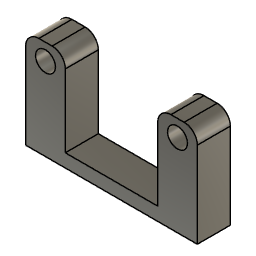
sumobot_base v24 (Autodesk Fusion 360 archive; units mm, degrees)
design "lidar_mount"
Autodesk Fusion 360 part; units mm, degrees
sketch "Sketch1" plane through (0, 0, 0) normal (0, 0, 1) x (1, 0, 0)
  line L0 (13, 2) -> (-13, 2)
  line L1 (-13, 2) -> (-13, -2)
  line L2 (-13, -2) -> (13, -2)
  line L3 (13, -2) -> (13, 2)
  line L4 (13, 2) -> (-13, -2) construction
  line L5 (-13, 2) -> (13, -2) construction
  dimension "d1" = 26
  dimension "d2" = 4
  constraint horizontal L0
  constraint perpendicular L0 L1
  constraint parallel L0 L2
  constraint parallel L1 L3
  constraint coincident L4 origin
  constraint coincident L5 origin
  measures "d1" distance of L1.end L2.end
  measures "d2" distance of L0.end L1.end
extrude "Extrude1" add sketch "Sketch1" along normal blind 2
sketch "Sketch2" plane through (0, 0, 2) normal (0, 0, 1) x (-1, 0, 0)
  line L0 (-13, 2) -> (-13, -2)
  line L1 (-13, -2) -> (13, -2)
  line L2 (13, -2) -> (13, 2)
  line L3 (13, 2) -> (-13, 2)
  line L4 (13, -2) -> (7, -2)
  line L5 (7, -2) -> (7, 2)
  line L6 (7, 2) -> (13, 2)
  line L7 (13, 2) -> (13, -2)
  line L8 (-13, -2) -> (-7, -2)
  line L9 (-7, -2) -> (-7, 2)
  line L10 (-7, 2) -> (-13, 2)
  line L11 (-13, 2) -> (-13, -2)
  constraint horizontal L4
  constraint vertical L5
  constraint horizontal L6
  constraint vertical L7
  constraint coincident L3 L5.end
  constraint coincident L1.end L2.start
  constraint horizontal L8
  constraint vertical L9
  constraint horizontal L10
  constraint vertical L11
  constraint coincident L3 L9.end
  constraint coincident L0.end L1.start
extrude "Extrude2" add sketch "Sketch2" along normal blind 13 contours L0 L1 L3 L8 L9 L10 L11 | L1 L2 L3 L4 L5 L6 L7
sketch "Sketch3" plane through (0, -2, 0) normal (0, -1, 0) x (1, 0, 0)
  line L0 (-13, 0) -> (13, 0)
  line L1 (13, 0) -> (13, 15)
  line L2 (13, 15) -> (7, 15)
  line L3 (7, 15) -> (7, 2)
  line L4 (7, 2) -> (-7, 2)
  line L5 (-7, 2) -> (-7, 15)
  line L6 (-7, 15) -> (-13, 15)
  line L7 (-13, 15) -> (-13, 0)
  circle A0 centre (-10, 12.5) radius 1.5
  circle A1 centre (10, 12.5) radius 1.5
  dimension "d7" = 3
  dimension "d8" = 3
  measures "d7" diameter of A0
  measures "d8" diameter of A1
extrude "Extrude3" cut sketch "Sketch3" against normal blind 5 contours A0 | A1
fillet "Fillet1" radius 2 4 edges at (-13, 0, 15) (-7, 0, 15) (7, 0, 15) (13, 0, 15)
extrude "Extrude4" add 1 faces at (-10.1113, -2, 4.3459) along direction (0, -1, 0) blind 1
sketch "Sketch4" plane through (0, 0, 2) normal (0, 0, 1) x (-1, 0, 0)
  line L0 (-7, 3) -> (-7, -2)
  line L1 (-7, -2) -> (7, -2)
  line L2 (7, -2) -> (7, 3)
  line L3 (7, 3) -> (-7, 3)
  circle A0 centre (4.5, 0.5) radius 1.5
  circle A1 centre (-4.5, 0.5) radius 1.5
extrude "Extrude5" cut sketch "Sketch4" against normal blind 2 contours A0 | A1
sketch "Sketch5" plane through (0, 0, 2) normal (0, 0, 1) x (-1, 0, 0)
  circle A0 centre (4.5, 0.5) radius 1.5
  circle A1 centre (-4.5, 0.5) radius 1.5
  line L0 (-7, 3) -> (-7, -2)
  line L1 (-7, -2) -> (7, -2)
  line L2 (7, -2) -> (7, 3)
  line L3 (7, 3) -> (-7, 3)
  circle A2 centre (4.5, 0.5) radius 1.5
  circle A3 centre (-4.5, 0.5) radius 1.5
  constraint concentric A0 A2
  constraint concentric A1 A3
extrude "Extrude6" add sketch "Sketch5" against normal blind 2 contours A0 A2 | A1 A3
